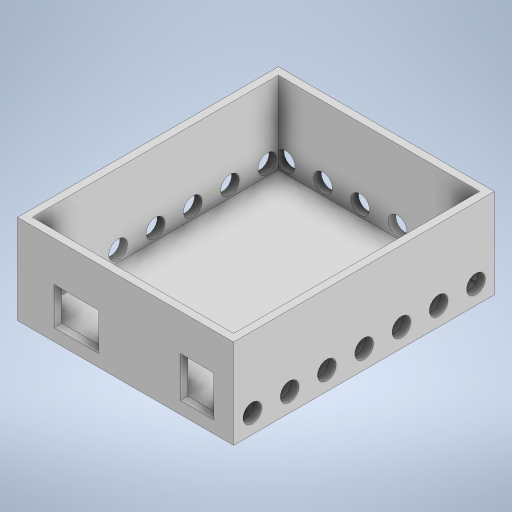
# Autodesk Inventor part: junction box
Saved by Autodesk Inventor 2024 (Build 280153000, 153)
## iProperties
Created: 2024-01-16
Part Number: junction box
Material: Generic
Document SubType Name: Modeling
Designer: ibrahm12
Density: 1 g/cm^3
Appearance: Default
Author: ibrahm12
Autodesk Inventor part; units mm, degrees
ref_plane "YZ Plane" through (0, 0, 0) normal (1, 0, 0) x (0, 1, 0)
ref_plane "XZ Plane" through (0, 0, 0) normal (0, 1, 0) x (-1, 0, 0)
ref_plane "XY Plane" through (0, 0, 0) normal (0, 0, 1) x (1, 0, 0)
sketch "Sketch1" plane through (0, 0, 0) normal (0, 1, 0) x (-1, 0, 0)
  point P0 (0, 0)
sketch "Sketch2" plane through (0, 0, 0) normal (0, 1, 0) x (-1, 0, 0)
  point P0 (0, 0)
sketch "Sketch3" plane through (0, 0, 0) normal (0, 1, 0) x (-1, 0, 0)
  line L0 (20.3143, 32.1) -> (-37.6857, 32.1)
  line L1 (-37.6857, 32.1) -> (-37.6857, -37.9)
  line L2 (-37.6857, -37.9) -> (20.3143, -37.9)
  line L3 (20.3143, -37.9) -> (20.3143, 32.1)
  point P0 (0, 0)
  dimension "d0" = 70
  dimension "d1" = 58
  constraints: 8 end point, 2 parallel, 1 horizontal, 1 perpendicular
  measures "d0" distance of L2.end L0.start
  measures "d1" distance of L0.start L0.end
extrude "Extrusion1" add sketch "Sketch3" along normal blind 24
sketch "Sketch4" plane through (0, 24, 0) normal (0, 1, 0) x (1, 0, 0)
  point P0 (0, 0)
sketch "Sketch5" plane through (0, 24, 0) normal (0, 1, 0) x (1, 0, 0)
  line L0 (-18.3143, 35.9) -> (35.6857, 35.9)
  line L1 (35.6857, 35.9) -> (35.6857, -30.1)
  line L2 (35.6857, -30.1) -> (-18.3143, -30.1)
  line L3 (-18.3143, -30.1) -> (-18.3143, 35.9)
  line L4 (37.6857, -32.1) -> (37.6857, 37.9) projected
  line L5 (-20.3143, -32.1) -> (37.6857, -32.1) projected
  line L6 (-20.3143, 37.9) -> (-20.3143, -32.1) projected
  line L7 (37.6857, 37.9) -> (-20.3143, 37.9) projected
  point P0 (0, 0)
  dimension "d4" = 2
  dimension "d5" = 2
  dimension "d6" = 2
  dimension "d7" = 2
  constraints: 8 end point, 2 parallel, 1 horizontal, 1 perpendicular
  measures "d4" distance between parallel lines of L4 L1
  measures "d5" distance between parallel lines of L5 L2
  measures "d6" distance between parallel lines of L6 L3
  measures "d7" distance between parallel lines of L0 L7
extrude "Extrusion2" cut sketch "Sketch5" against normal blind 22 contours L0 L1 L2 L3
sketch "Sketch6" plane through (-20.3143, 0, 32.1) normal (0, 0, 1) x (1, 0, 0)
  line L0 (9.8, 13.3) -> (21.8, 13.3)
  line L1 (21.8, 13.3) -> (21.8, 3.3)
  line L2 (21.8, 3.3) -> (9.8, 3.3)
  line L3 (9.8, 3.3) -> (9.8, 13.3)
  line L4 (0, 0) -> (0, 24) projected
  line L5 (0, 0) -> (58, 0) projected
  point P0 (20.3143, 0)
  dimension "d10" = 9.8
  dimension "d11" = 12
  dimension "d12" = 10
  dimension "d13" = 3.3
  constraints: 8 end point, 2 parallel, 1 horizontal, 1 perpendicular
  measures "d10" distance between parallel lines of L4 L3
  measures "d11" distance of L1.end L2.end
  measures "d12" distance of L2.end L0.start
  measures "d13" distance between parallel lines of L5 L2
extrude "Extrusion3" cut sketch "Sketch6" against normal blind 22.45
sketch "Sketch7" plane through (-20.3143, 0, 32.1) normal (0, 0, 1) x (1, 0, 0)
  line L0 (43.7, 14.2) -> (52.7, 14.2)
  line L1 (52.7, 14.2) -> (52.7, 3.3)
  line L2 (52.7, 3.3) -> (43.7, 3.3)
  line L3 (43.7, 3.3) -> (43.7, 14.2)
  line L4 (58, 0) -> (58, 24) projected
  line L5 (0, 0) -> (58, 0) projected
  point P0 (20.3143, 0)
  dimension "d16" = 5.3
  dimension "d17" = 9
  dimension "d18" = 10.9
  dimension "d19" = 3.3
  constraints: 8 end point, 2 parallel, 1 horizontal, 1 perpendicular
  measures "d16" distance between parallel lines of L4 L1
  measures "d17" distance of L0.start L0.end
  measures "d18" distance of L2.end L0.start
  measures "d19" distance between parallel lines of L5 L2
extrude "Extrusion4" cut sketch "Sketch7" against normal blind 25.175
sketch "Sketch8" plane through (-20.3143, 0, -37.9) normal (-1, 0, 0) x (0, 0, 1)
  circle A0 centre (65, 5) radius 2.5
  line L0 (0, 0) -> (70, 0) projected
  line L1 (70, 0) -> (70, 24) projected
  circle A1 centre (55, 5) radius 2.5
  circle A2 centre (45, 5) radius 2.5
  circle A3 centre (35, 5) radius 2.5
  circle A4 centre (25, 5) radius 2.5
  circle A5 centre (15, 5) radius 2.5
  circle A6 centre (5, 5) radius 2.5
  point P0 (37.9, 0)
  point P1 (35, 0)
  dimension "d22" = 5
  dimension "d23" = 5
  dimension "d24" = 5
  dimension "d25" = 5
  dimension "d26" = 10
  dimension "d27" = 5
  dimension "d28" = 5
  dimension "d29" = 5
  dimension "d30" = 10
  dimension "d31" = 5
  dimension "d32" = 10
  dimension "d33" = 5
  dimension "d34" = 5
  dimension "d35" = 10
  dimension "d36" = 5
  dimension "d37" = 5
  dimension "d38" = 5
  dimension "d39" = 10
  dimension "d40" = 5
  dimension "d41" = 10
  dimension "d42" = 5
  constraints: 7 centre point, 1 midpoint
  measures "d22" diameter of A0
  measures "d23" distance from line of L0 A0.centre
  measures "d24" distance from line of A0.centre L1
  measures "d25" diameter of A1
  measures "d26" distance of A0.centre A1.centre
  measures "d27" distance from line of L0 A1.centre
  measures "d28" diameter of A2
  measures "d29" distance from line of L0 A2.centre
  measures "d30" distance of A1.centre A2.centre
  measures "d31" diameter of A3
  measures "d32" distance of A2.centre A3.centre
  measures "d33" distance of point (35, 0) A3.centre
  measures "d34" diameter of A4
  measures "d35" distance of A3.centre A4.centre
  measures "d36" diameter of A5
  measures "d37" distance from line of L0 A4.centre
  measures "d38" distance from line of L0 A5.centre
  measures "d39" distance of A5.centre A4.centre
  measures "d40" diameter of A6
  measures "d41" distance of A5.centre A6.centre
  measures "d42" distance from line of L0 A6.centre
extrude "Extrusion5" cut sketch "Sketch8" against normal blind 44.225
sketch "Sketch9" plane through (-20.3143, 0, -37.9) normal (-1, 0, 0) x (0, 0, 1)
  point P0 (37.9, 0)
sketch "Sketch10" plane through (37.6857, 0, 32.1) normal (1, 0, 0) x (0, 0, -1)
  circle A0 centre (5, 5.0214) radius 2.5
  line L0 (0, 0) -> (0, 24) projected
  circle A1 centre (15, 5) radius 2.5
  line L1 (0, 0) -> (70, 0) projected
  circle A2 centre (25, 5) radius 2.5
  circle A3 centre (35, 5) radius 2.5
  circle A4 centre (45, 5) radius 2.5
  circle A5 centre (55, 5) radius 2.5
  circle A6 centre (65, 5) radius 2.5
  point P0 (32.1, 0)
  dimension "d45" = 5
  dimension "d46" = 5
  dimension "d47" = 5
  dimension "d48" = 10
  dimension "d49" = 5
  dimension "d50" = 5
  dimension "d51" = 5
  dimension "d52" = 10
  dimension "d53" = 5
  dimension "d54" = 5
  dimension "d55" = 10
  dimension "d56" = 5
  dimension "d57" = 10
  dimension "d58" = 5
  dimension "d59" = 5
  dimension "d60" = 5
  dimension "d61" = 10
  dimension "d62" = 5
  dimension "d63" = 10
  dimension "d64" = 5
  constraints: 7 centre point
  measures "d45" diameter of A0
  measures "d46" distance from line of L0 A0.centre
  measures "d47" diameter of A1
  measures "d48" horizontal distance of A0.centre A1.centre
  measures "d49" distance from line of L1 A1.centre
  measures "d50" diameter of A2
  measures "d51" distance from line of L1 A2.centre
  measures "d52" distance of A1.centre A2.centre
  measures "d53" diameter of A3
  measures "d54" distance from line of L1 A3.centre
  measures "d55" distance of A2.centre A3.centre
  measures "d56" diameter of A4
  measures "d57" distance of A3.centre A4.centre
  measures "d58" distance from line of L1 A4.centre
  measures "d59" diameter of A5
  measures "d60" distance from line of L1 A5.centre
  measures "d61" distance of A4.centre A5.centre
  measures "d62" diameter of A6
  measures "d63" distance of A5.centre A6.centre
  measures "d64" distance from line of L1 A6.centre
extrude "Extrusion6" cut sketch "Sketch10" against normal blind 41.5
sketch "Sketch11" plane through (37.6857, 0, -37.9) normal (0, 0, -1) x (-1, 0, 0)
  circle A0 centre (4, 5) radius 2.5
  line L0 (0, 0) -> (0, 24) projected
  line L1 (0, 0) -> (58, 0) projected
  circle A1 centre (14, 5) radius 2.5
  circle A2 centre (24, 5) radius 2.5
  circle A3 centre (34, 5) radius 2.5
  circle A4 centre (44, 5) radius 2.5
  circle A5 centre (54, 5) radius 2.5
  point P0 (37.6857, 0)
  dimension "d67" = 5
  dimension "d68" = 4
  dimension "d69" = 5
  dimension "d70" = 5
  dimension "d71" = 10
  dimension "d72" = 5
  dimension "d73" = 5
  dimension "d74" = 10
  dimension "d75" = 5
  dimension "d76" = 5
  dimension "d77" = 10
  dimension "d78" = 5
  dimension "d79" = 5
  dimension "d80" = 10
  dimension "d81" = 5
  dimension "d82" = 5
  dimension "d83" = 10
  dimension "d84" = 5
  constraints: 6 centre point
  measures "d67" diameter of A0
  measures "d68" distance from line of L0 A0.centre
  measures "d69" distance from line of L1 A0.centre
  measures "d70" diameter of A1
  measures "d71" distance of A1.centre A0.centre
  measures "d72" distance from line of L1 A1.centre
  measures "d73" diameter of A2
  measures "d74" distance of A1.centre A2.centre
  measures "d75" distance from line of L1 A2.centre
  measures "d76" diameter of A3
  measures "d77" distance of A2.centre A3.centre
  measures "d78" distance from line of L1 A3.centre
  measures "d79" diameter of A4
  measures "d80" distance of A3.centre A4.centre
  measures "d81" distance from line of L1 A4.centre
  measures "d82" diameter of A5
  measures "d83" distance of A4.centre A5.centre
  measures "d84" distance from line of L1 A5.centre
extrude "Extrusion7" cut sketch "Sketch11" against normal blind 2
body "Solid1"
